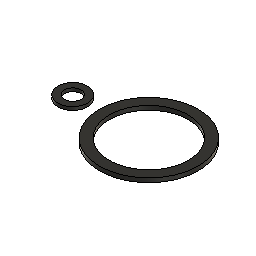
Spacers (Autodesk Fusion 360 design; units mm, degrees)
Autodesk Fusion 360 part; units mm, degrees
sketch "Sketch1" plane through (0, 0, 0) normal (0, 0, 1) x (1, 0, 0)
  circle A0 centre (0, 0) radius 3.9688
  circle A1 centre (0, 0) radius 7.1437
  dimension "d1" = 7.9375
  dimension "d2" = 3.175
  constraint coincident A0.centre A1.centre
  measures "d1" diameter of A0
extrude "Extrude1" add sketch "Sketch1" along normal blind 1.5875 makes body 1
sketch "Sketch2" plane through (0, 0, 0) normal (0, 0, 1) x (1, 0, 0)
  circle A0 centre (36.824, -0.0529) radius 19.05
  circle A1 centre (36.824, -0.0529) radius 23.8125
  dimension "d5" = 38.1
  dimension "d6" = 4.7625
  measures "d5" diameter of A0
extrude "Extrude2" add sketch "Sketch2" along normal blind 2 separate body makes body 2
equation "d1 = ( 5 / 16 ) * 1 in"
equation "d2 = ( 1 / 8 ) * 1 in"
equation "d3 = ( 1 / 16 ) * 1 in"
equation "d6 = ( 3 / 16 ) * 1 in"
named bodies: "Spacer1", "Spacer2"
